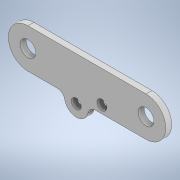
# Autodesk Inventor part: ramie_1_wahacza
Saved by Autodesk Inventor 2020.3 (Build 243373000, 373)
## iProperties
Created: 2021-10-24
Part Number: ramie_1_wahacza
Material: Ogólny
Document SubType Name: Modeling
Designer: patry
Density: 1 g/cm^3
Appearance: Domyślna
Author: patry
Autodesk Inventor part; units mm, degrees
ref_plane "YZ Plane" through (0, 0, 0) normal (1, 0, 0) x (0, 1, 0)
ref_plane "XZ Plane" through (0, 0, 0) normal (0, 1, 0) x (-1, 0, 0)
ref_plane "XY Plane" through (0, 0, 0) normal (0, 0, 1) x (1, 0, 0)
sketch "Szkic1" plane through (0, 0, 0) normal (0, 0, 1) x (1, 0, 0)
  line L0 (0, 0) -> (60, 0) construction
  line L1 (0, -10) -> (14.7824, -10)
  line L2 (60, 10) -> (0, 10)
  arc A0 (0, 10) -> (0, -10) centre (0, 0) ccw
  arc A1 (60, -10) -> (60, 10) centre (60, 0) ccw
  arc A2 (30.2373, -10) -> (18.9235, -10) centre (24.5804, -12) ccw construction
  arc A3 (18.7016, -13.2) -> (30.4592, -13.2) centre (24.5804, -12) ccw
  line L3 (34.3784, -10) -> (60, -10)
  line L4 (18.9235, -10) -> (30.2373, -10)
  arc A4 (34.3784, -10) -> (30.4592, -13.2) centre (34.3784, -14) ccw
  arc A5 (18.7016, -13.2) -> (14.7824, -10) centre (14.7824, -14) ccw
  point P0 (30, 0)
  point P1 (37.5804, -6)
  point P2 (29.5804, -5)
  dimension "d0" = 60
  dimension "d1" = 20
  dimension "d20" = 12
  dimension "d21" = 4
  dimension "d22" = 13
  dimension "d23" = 6
  dimension "d24" = 30
  dimension "d25" = 1
  dimension "d26" = 8
  dimension "d27" = 5
  constraints: 14 point on circle, 12 end point, 12 tangent, 6 centre point, 3 coincident, 3 parallel, 2 point on line, 1 equal radius, 1 horizontal, 1 midpoint
  measures "d0" distance of L0.start L0.end
  measures "d1" diameter of A1
  measures "d20" diameter of A2
  measures "d21" radius of A4
  measures "d22" horizontal distance of point (37.58, -6) point (24.58, -12)
  measures "d23" vertical distance of point (37.58, -6) point (24.58, -12)
  measures "d24" distance of point (29.58, -5) point (0, 0)
  measures "d25" vertical distance of point (37.58, -6) point (29.58, -5)
  measures "d26" horizontal distance of point (37.58, -6) point (29.58, -5)
  measures "d27" distance from line of L1 point (29.58, -5)
extrude "Wyciągnięcie proste1" add sketch "Szkic1" along normal blind 3
hole "Otwór1" at (0, 0, 0) at (60, 0, 0) direction (0, 0, 1) diameter 8 end through all
hole "Otwór2" at (37.5804, -6, 0) at (24.5804, -12, 0) direction (0, 0, 1) diameter 5 end through all
